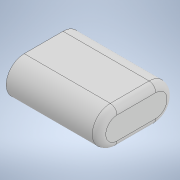
# Autodesk Inventor part: Among Us Goggles
Saved by Autodesk Inventor 2022 (Build 260153000, 153)
## iProperties
Created: 2021-10-11
Part Number: Among Us Goggles
Material: Generic
Document SubType Name: Modeling
Designer: Vineeth
Density: 1 g/cm^3
Appearance: Default
Author: Vineeth
Autodesk Inventor part; units mm, degrees
ref_plane "YZ Plane" through (0, 0, 0) normal (1, 0, 0) x (0, 1, 0)
ref_plane "XZ Plane" through (0, 0, 0) normal (0, 1, 0) x (-1, 0, 0)
ref_plane "XY Plane" through (0, 0, 0) normal (0, 0, 1) x (1, 0, 0)
sketch "Sketch1" plane through (0, 0, 0) normal (1, 0, 0) x (0, 1, 0)
  line L0 (0, 0) -> (0, -44.3) construction
  line L1 (10.65, -10.65) -> (10.65, -33.65)
  line L2 (-10.65, -33.65) -> (-10.65, -10.65)
  arc A0 (10.65, -10.65) -> (-10.65, -10.65) centre (0, -10.65) ccw
  arc A1 (-10.65, -33.65) -> (10.65, -33.65) centre (0, -33.65) ccw
  point P0 (0, -22.15)
  dimension "d0" = 44.3
  dimension "d1" = 21.3
  constraints: 8 end point, 6 point on circle, 4 tangent, 2 centre point, 2 point on line, 1 midpoint, 1 parallel, 1 vertical
  measures "d0" distance of L0.start L0.end
  measures "d1" distance between parallel lines of L2 L1
extrude "Extrusion1" add sketch "Sketch1" against normal blind 55
fillet "Fillet1" radius 4 4 edges at (0, 0, 0) (0, -10.65, -22.15) (0, 0, -44.3) (0, 10.65, -22.15)
body "Solid1"
